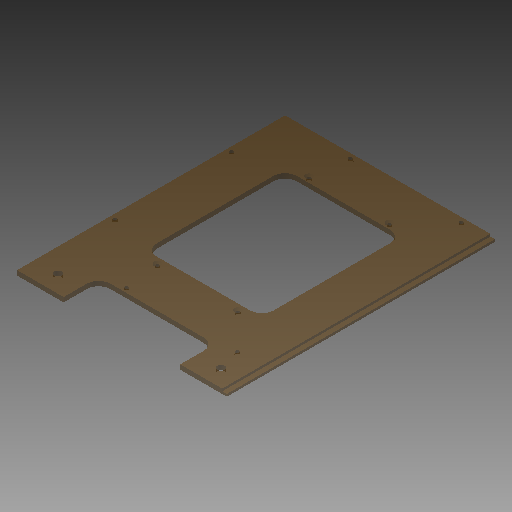
# Autodesk Inventor part: Boden
Saved by Autodesk Inventor 2018 (Build 220112000, 112)
## iProperties
Created: 2013-02-21
Part Number: Boden
Material: Polycarbonate, Smoke
Document SubType Name: Modeling
Designer: Neef
Mass: 196.203 g
Surface Area: 860.962 cm^2
Volume: 163.503 cm^3
Density: 1.2 g/cm^3
Appearance: Polycarbonate - Smoked
Author: Neef
Autodesk Inventor part; units mm, degrees
ref_plane "YZ Plane" through (0, 0, 0) normal (1, 0, 0) x (0, 1, 0)
ref_plane "XZ Plane" through (0, 0, 0) normal (0, 1, 0) x (-1, 0, 0)
ref_plane "XY Plane" through (0, 0, 0) normal (0, 0, 1) x (1, 0, 0)
sketch "Skizze1" plane through (0, 0, 0) normal (0, 0, 1) x (1, 0, 0)
  line L0 (0, 161) -> (0, -161) projected
  line L1 (-126, 0) -> (126, 0) projected
  line L2 (-90, 115) -> (90, 115)
  line L3 (90, 115) -> (90, -115)
  line L4 (90, -115) -> (-90, -115)
  line L5 (-90, -115) -> (-90, 115)
  point P0 (0, 0)
  point P1 (0, 115)
  point P2 (-90, 0)
  dimension "d0" = 230
  dimension "d1" = 180
  constraints: 8 end point, 2 midpoint, 2 parallel, 2 point on line, 1 horizontal, 1 perpendicular
  measures "d0" distance of L4.end L2.start
  measures "d1" distance of L2.start L2.end
extrude "Extrusion1" add sketch "Skizze1" along normal blind 4
sketch "Skizze2" plane through (0, 0, 4) normal (0, 0, 1) x (1, 0, 0)
  line L0 (-90, -115) -> (-90, 115) projected
  line L1 (90, -115) -> (-90, -115) projected
  line L2 (90, 115) -> (90, -115) projected
  point P0 (0, 0)
  point P1 (-70, -100)
  point P2 (70, -100)
  dimension "d4" = 20
  dimension "d5" = 20
  dimension "d6" = 15
  dimension "d7" = 15
  measures "d4" distance from line of L0 point (-70, -100)
  measures "d5" distance from line of L2 point (70, -100)
  measures "d6" distance from line of L1 point (-70, -100)
  measures "d7" distance from line of L1 point (70, -100)
hole "Bohrung1" at (-70, -100, 4) at (70, -100, 4) direction (0, 0, -1) diameter 6.4 end through all
sketch "Skizze3" plane through (0, 0, 4) normal (0, 0, 1) x (1, 0, 0)
  line L0 (90, -115) -> (-90, -115) projected
  line L1 (90, 115) -> (90, -115) projected
  line L2 (90, 115) -> (86, 115)
  line L3 (86, 115) -> (86, -115)
  line L4 (86, -115) -> (90, -115)
  line L5 (90, -115) -> (90, 115)
  point P0 (0, 0)
  dimension "d15" = 4
  constraints: 8 end point, 2 parallel, 1 horizontal, 1 perpendicular, 1 point on line
  measures "d15" distance between parallel lines of L5 L3
extrude "Extrusion2" cut sketch "Skizze3" against normal blind 2
sketch "Skizze4" plane through (0, 0, 4) normal (0, 0, 1) x (1, 0, 0)
  line L0 (-90, 115) -> (86, 115) projected
  line L1 (-90, -115) -> (-90, 115) projected
  line L2 (-50, 75) -> (50, 75)
  line L3 (50, 75) -> (50, -45)
  line L4 (50, -45) -> (-50, -45)
  line L5 (-50, -45) -> (-50, 75)
  point P0 (0, 0)
  dimension "d18" = 100
  dimension "d19" = 120
  dimension "d20" = 40
  dimension "d21" = 40
  constraints: 8 end point, 2 parallel, 1 horizontal, 1 perpendicular
  measures "d18" distance of L2.start L2.end
  measures "d19" distance of L4.end L2.start
  measures "d20" distance between parallel lines of L1 L5
  measures "d21" distance between parallel lines of L0 L2
extrude "Extrusion3" cut sketch "Skizze4" against normal through all
fillet "Rundung1" radius 10 4 edges at (-50, 75, 2) (50, 75, 2) (50, -45, 2) (-50, -45, 2)
sketch "Skizze5" plane through (0, 0, 4) normal (0, 0, 1) x (1, 0, 0)
  line L0 (-90, -115) -> (-90, 115) projected
  line L1 (86, -115) -> (-90, -115) projected
  line L2 (-50, -115) -> (50, -115)
  line L3 (50, -115) -> (50, -85)
  line L4 (50, -85) -> (-50, -85)
  line L5 (-50, -85) -> (-50, -115)
  point P0 (0, 0)
  dimension "d25" = 100
  dimension "d26" = 30
  dimension "d27" = 40
  constraints: 8 end point, 2 parallel, 1 horizontal, 1 perpendicular, 1 point on line
  measures "d25" distance of L3.end L4.end
  measures "d26" distance of L4.end L2.start
  measures "d27" distance between parallel lines of L0 L5
extrude "Extrusion4" cut sketch "Skizze5" against normal through all
fillet "Rundung2" radius 10 2 edges at (-50, -85, 2) (50, -85, 2)
sketch "Skizze6" plane through (0, 0, 0) normal (0, 0, -1) x (-1, 0, 0)
  line L0 (90, -115) -> (50, -115) projected
  line L1 (90, 115) -> (90, -115) projected
  line L2 (-90, 115) -> (90, 115) projected
  line L3 (-90, -115) -> (-90, 115) projected
  line L4 (-40, -85) -> (40, -85) projected
  point P0 (0, 0)
  point P1 (-65, 111)
  point P2 (30, 111)
  point P3 (86, 65)
  point P4 (86, -35)
  point P5 (30, -81)
  point P6 (-65, -81)
  dimension "d31" = 60
  dimension "d32" = 4
  dimension "d33" = 25
  dimension "d34" = 50
  dimension "d35" = 4
  dimension "d36" = 4
  dimension "d37" = 80
  dimension "d38" = 4
  dimension "d39" = 60
  dimension "d40" = 4
  dimension "d41" = 25
  dimension "d42" = 4
  measures "d31" distance from line of L1 point (30, 111)
  measures "d32" distance from line of L2 point (30, 111)
  measures "d33" distance from line of L3 point (-65, 111)
  measures "d34" distance from line of L2 point (86, 65)
  measures "d35" distance from line of L1 point (86, 65)
  measures "d36" distance from line of L2 point (-65, 111)
  measures "d37" distance from line of point (86, -35) L0
  measures "d38" distance from line of L1 point (86, -35)
  measures "d39" distance from line of L1 point (30, -81)
  measures "d40" distance from line of point (30, -81) L4
  measures "d41" distance from line of L3 point (-65, -81)
  measures "d42" distance from line of L4 point (-65, -81)
hole "Bohrung2" at (65, 111, 0) at (-30, 111, 0) at (-86, 65, 0) at (-86, -35, 0) at (-30, -81, 0) at (65, -81, 0) direction (0, 0, 1) diameter 3.2 end through all countersink diameter 6.2 countersink angle 90
sketch "Skizze7" plane through (0, 0, 4) normal (0, 0, 1) x (1, 0, 0)
  line L0 (-49.5, 75) -> (-49.5, 85) projected
  line L1 (49.5, 85) -> (-49.5, 85) projected
  line L2 (49.5, 85) -> (49.5, 75) projected
  line L3 (49.5, 75) -> (-49.5, 75) projected
  circle A0 centre (-34.5, 80) radius 1.2295 projected
  circle A1 centre (34.5, 80) radius 1.2295 projected
  circle A2 centre (34.5, -50) radius 1.2295 projected
  circle A3 centre (-34.5, -50) radius 1.2295 projected
  line L4 (-49.5, -45) -> (-49.5, -55) projected
  line L5 (49.5, -55) -> (-49.5, -55) projected
  line L6 (49.5, -55) -> (49.5, -45) projected
  line L7 (49.5, -45) -> (-49.5, -45) projected
  point P0 (0, 0)
  constraints: 4 coincident
hole "Bohrung3" at (-34.5, -50, 4) at (34.5, -50, 4) at (34.5, 80, 4) at (-34.5, 80, 4) direction (0, 0, -1) diameter 3.2 end through all countersink diameter 6.2 countersink angle 90
equation "\"d5\" = d4"
equation "\"d7\" = d6"
equation "\"d35\" = d32"
equation "\"d36\" = d32"
equation "\"d38\" = d35"
equation "\"d40\" = d38"
equation "\"d41\" = d33"
equation "\"d42\" = d40"
